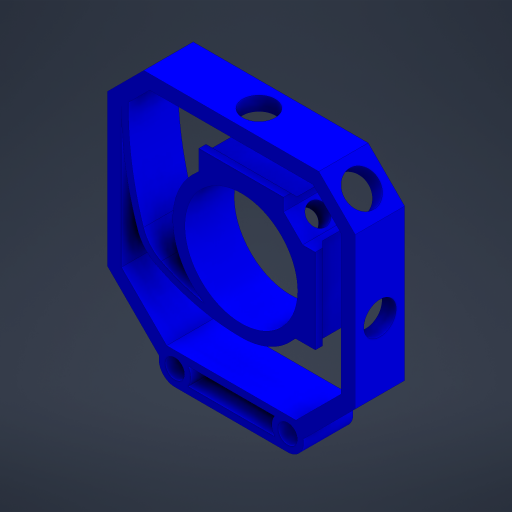
# Autodesk Inventor part: Laser Holder (USB)
Saved by Autodesk Inventor 2023.4 (Build 274418000, 418)
## iProperties
Created: 2022-07-25
Part Number: Laser Holder (USB)
Material: Generic
Document SubType Name: Modeling
Designer: xSibe
Density: 1 g/cm^3
Appearance: Plastic Blue
Author: xSibe
Autodesk Inventor part; units mm, degrees
ref_plane "YZ Plane" through (0, 0, 0) normal (1, 0, 0) x (0, 1, 0)
ref_plane "XZ Plane" through (0, 0, 0) normal (0, 1, 0) x (-1, 0, 0)
ref_plane "XY Plane" through (0, 0, 0) normal (0, 0, 1) x (1, 0, 0)
sketch "Sketch1" plane through (0, 0, 0) normal (0, 0, 1) x (1, 0, 0)
  circle A0 centre (10, 3.85) radius 1.5625 projected
  circle A1 centre (-10, 3.85) radius 1.5625 projected
  line L0 (-16.9, 0) -> (16.9, 0) projected
  line L1 (16.9, 0) -> (16.9, 7.7) projected
  line L2 (-16.9, 7.7) -> (16.9, 7.7) projected
  line L3 (-16.9, 0) -> (-16.9, 7.7) projected
  circle A2 centre (-10, 3.85) radius 2.8125
  circle A3 centre (10, 3.85) radius 2.8125
  line L4 (-10, 6.6625) -> (10, 6.6625)
  line L5 (10, 1.0375) -> (-10, 1.0375)
  line L6 (-10, 2.2875) -> (10, 2.2875)
  line L7 (-10, 5.4125) -> (10, 5.4125)
  line L8 (-17.05, 7.7) -> (-17.05, 42.1) projected
  line L9 (17.05, 7.7) -> (17.05, 42.1) projected
  line L10 (-17.05, 24.9) -> (17.05, 24.9)
  line L11 (0, 24.9) -> (1.7678, 26.6678)
  line L12 (0, 24.9) -> (2.5, 24.9) construction
  circle A4 centre (1.7678, 26.6678) radius 10
  circle A5 centre (1.7678, 26.6678) radius 7.5
  circle A6 centre (1.7678, 26.6678) radius 12.125
  line L13 (1.7678, 26.6678) -> (1.7678, 38.7928)
  line L14 (1.7678, 38.7928) -> (1.7678, 37.7928)
  line L15 (-5.7322, 35.7928) -> (9.2678, 35.7928)
  line L16 (9.2678, 35.7928) -> (9.2678, 39.7928)
  line L17 (9.2678, 39.7928) -> (-5.7322, 39.7928)
  line L18 (-5.7322, 39.7928) -> (-5.7322, 35.7928)
  line L19 (-5.7322, 35.7928) -> (9.2678, 39.7928) construction
  line L20 (9.2678, 35.7928) -> (-5.7322, 39.7928) construction
  line L21 (1.7678, 26.6678) -> (10.3414, 35.2414)
  line L22 (10.3414, 35.2414) -> (9.8995, 34.7995)
  line L23 (12.7279, 34.0924) -> (9.1924, 37.6279)
  line L24 (9.1924, 37.6279) -> (7.0711, 35.5066)
  line L25 (7.0711, 35.5066) -> (10.6066, 31.9711)
  line L26 (10.6066, 31.9711) -> (12.7279, 34.0924)
  line L27 (12.7279, 34.0924) -> (7.0711, 35.5066) construction
  line L28 (9.1924, 37.6279) -> (10.6066, 31.9711) construction
  line L29 (12.7279, 34.0924) -> (17.7279, 34.0924) construction
  line L30 (10.8928, 19.1678) -> (10.8928, 34.1678)
  line L31 (10.8928, 34.1678) -> (14.8928, 34.1678)
  line L32 (14.8928, 34.1678) -> (14.8928, 19.1678)
  line L33 (14.8928, 19.1678) -> (10.8928, 19.1678)
  line L34 (1.7678, 38.7928) -> (1.7678, 40.7928)
  line L35 (14.8928, 26.6678) -> (16.8928, 26.6678)
  line L36 (-10.2178, 5.4322) -> (10.2178, 5.4322)
  line L37 (19.4678, 14.6822) -> (19.4678, 39.3678)
  line L38 (14.4678, 44.3678) -> (-14.4678, 44.3678)
  line L39 (-19.4678, 39.3678) -> (-19.4678, 14.6822)
  line L40 (-19.4678, 5.4322) -> (19.4678, 44.3678) construction
  line L41 (19.4678, 5.4322) -> (-19.4678, 44.3678) construction
  line L42 (-10.2178, 5.4322) -> (-19.4678, 14.6822)
  line L43 (10.2178, 5.4322) -> (19.4678, 14.6822)
  line L44 (14.4678, 44.3678) -> (19.4678, 39.3678)
  line L45 (-14.4678, 44.3678) -> (-19.4678, 39.3678)
  line L46 (-15.5033, 46.8678) -> (-21.9678, 40.4033)
  line L47 (-21.9678, 40.4033) -> (-21.9678, 13.6467)
  line L48 (-21.9678, 13.6467) -> (-11.2533, 2.9322)
  line L49 (-11.2533, 2.9322) -> (11.2533, 2.9322)
  line L50 (11.2533, 2.9322) -> (21.9678, 13.6467)
  line L51 (21.9678, 13.6467) -> (21.9678, 40.4033)
  line L52 (21.9678, 40.4033) -> (15.5033, 46.8678)
  line L53 (15.5033, 46.8678) -> (-15.5033, 46.8678)
  circle A7 centre (-10, 3.85) radius 1.705
  circle A8 centre (10, 3.85) radius 1.707
  line L54 (1.7678, 14.5428) -> (-15.7322, 14.5428)
  line L55 (-15.7322, 14.5428) -> (-15.7322, 19.5428)
  arc A9 (-15.7322, 19.5428) -> (1.7678, 14.5428) centre (1.7678, 47.6678) ccw
  arc A10 (-19.4678, 39.3678) -> (-15.7322, 19.5428) centre (35.007, 39.3678) ccw
  arc A11 (-18.2027, 40.6328) -> (-14.7184, 20.3874) centre (35.007, 39.3678) ccw
  arc A12 (-14.7184, 20.3874) -> (-4.8026, 16.4773) centre (1.7678, 47.6678) ccw
  line L56 (-14.7184, 20.3874) -> (-15.5549, 22.7433)
  line L57 (-15.7322, 19.5428) -> (-16.5884, 21.8916)
  arc A13 (-15.5549, 22.7433) -> (-12.4238, 19.1263) centre (-9.6619, 24.6809) ccw
  arc A14 (-16.5884, 21.8916) -> (-13.459, 18.2499) centre (-10.5081, 23.9511) ccw
  line L58 (-10, 6.6625) -> (-11.448, 6.6625)
  line L59 (10, 6.6625) -> (11.448, 6.6625)
  point P0 (0, 0)
  point P1 (-7.6615, 2.2875)
  point P2 (-7.6615, 5.4125)
  point P3 (7.6615, 5.4125)
  point P4 (7.6615, 2.2875)
  point P5 (7.3415, 2.9322)
  point P6 (-7.3415, 2.9322)
  point P7 (-11.1858, 6.4003)
  point P8 (11.1858, 6.4003)
  point P9 (-5.7322, 36.1949)
  point P10 (11.2949, 19.1678)
  point P11 (11.2949, 34.1678)
  point P12 (11.925, 33.2894)
  point P13 (8.3894, 36.825)
  point P14 (9.2678, 36.1949)
  point P15 (12.7519, 4.4308)
  point P16 (-12.7519, 4.4308)
  point P17 (7.3572, 35.7928)
  point P18 (10.8928, 32.2572)
  point P19 (13.8928, 26.6678)
  point P20 (12.5533, 33.9178)
  point P21 (9.0178, 37.4533)
  point P22 (1.7678, 38.7928)
  point P23 (10.3414, 35.2414)
  point P24 (12.6525, 34.1678)
  point P25 (9.2678, 37.5525)
  point P26 (-5.6062, 36.2928)
  point P27 (11.3928, 19.2938)
  point P28 (11.3928, 34.0417)
  point P29 (9.1417, 36.2928)
  dimension "d0" = 1.25
  dimension "d1" = 1.25
  dimension "d2" = 2.5
  dimension "d3" = 45
  dimension "d4" = 20
  dimension "d5" = 2.5
  dimension "d6" = 2.125
  dimension "d7" = 1
  dimension "d8" = 15
  dimension "d9" = 4
  dimension "d10" = 0.625
  dimension "d11" = 5
  dimension "d12" = 135
  dimension "d13" = 3
  dimension "d14" = 2
  dimension "d15" = 2
  dimension "d16" = 38.9355
  dimension "d17" = 38.9355
  dimension "d18" = 9.25
  dimension "d19" = 9.25
  dimension "d20" = 9.25
  dimension "d21" = 9.25
  dimension "d22" = 5
  dimension "d23" = 5
  dimension "d24" = 5
  dimension "d25" = 5
  dimension "d26" = 2.5
  dimension "d46" = 0.1425
  dimension "d47" = 0.1445
  dimension "d48" = 17.5
  dimension "d49" = 5
  dimension "d50" = 1.25
  dimension "d51" = 2.5
  dimension "d52" = 2.5
  constraints: 108 end point, 29 point on circle, 18 point on line, 13 centre point, 13 tangent, 10 midpoint, 8 parallel, 7 horizontal, 7 perpendicular, 4 symmetric about line, 2 equal length, 1 coincident, 1 vertical, 8 other
  measures "d0" radial gap between concentric circles of A1 A2
  measures "d1" radial gap between concentric circles of A0 A3
  measures "d2" distance of L11.start L11.end
  measures "d3" angle of L12 L11
  measures "d4" diameter of A4
  measures "d5" radial gap between concentric circles of A4 A5
  measures "d6" radial gap between concentric circles of A4 A6
  measures "d7" distance of L13.end L14.end
  measures "d8" distance of L17.end L16.end
  measures "d9" distance of L16.end L15.end
  measures "d10" distance of L21.end L22.end
  measures "d11" distance of L23.start L23.end
  measures "d12" angle of L29 L23
  measures "d13" distance of L24.end L23.end
  measures "d14" distance of L13.end L34.end
  measures "d15" distance of L35.start L35.end
  measures "d16" distance of L40.end L41.end
  measures "d17" distance of L41.end L40.start
  measures "d18" distance of L36.start L40.start
  measures "d19" distance of L39.end L40.start
  measures "d20" distance of L36.end L41.start
  measures "d21" distance of L37.start L41.start
  measures "d22" distance of L38.start L40.end
  measures "d23" distance of L37.end L40.end
  measures "d24" distance of L38.end L41.end
  measures "d25" distance of L39.start L41.end
  measures "d26" distance between parallel lines of L38 L53
  measures "d46" radial gap between concentric circles of A1 A7
  measures "d47" radial gap between concentric circles of A0 A8
  measures "d48" distance of L54.start L54.end
  measures "d49" distance of L54.end L55.end
  measures "d50" radial gap between concentric circles of A10 A11
  measures "d51" distance of L56.start L56.end
  measures "d52" distance of L55.end L57.end
extrude "Extrusion1" add sketch "Sketch1" along normal mid plane 8.75 contours A8 L49 A3 L7 | L7 A3 L36 A8 | A8 L43 A3 L50 | L50 A3 L6 A8 | A8 L6 A3 L49 | L7 A2 L36 A3 | L36 A3 L43 A8 | A3 L43 L2 L50 | L36 A2 L4 A3 | L7 A7 L36 A2 | A2 L49 A7 L7 | A3 L5 A2 L6 | A3 L59 L43 | L2 L43 L9 L50 | A2 L6 A7 L49 | L36 A7 L42 A2 | A2 L48 A7 L6 | L9 L43 L37 L44 L38 L45 L39 L42 L8 L48 L47 L46 L53 L52 L51 L50 | A2 L42 L58 | L42 A2 L48 L2 | L2 L48 L8 L42 | L42 A7 L48 A2 | A10 L45 A11 L8 | L8 L10 A11 A12 A6 A9 A14 A10 | L32 L33 A6 L10 | L10 A6 L26 L23 L31 L32 | L8 A11 L10 | A6 L33 L30 A4 L10 | L10 A4 L30 L26 A6 | A13 A12 L56 | A6 L10 A4 L30 L33 | A6 L18 L15 A4 L10 | L56 A11 | L26 L30 L31 A6 | A6 L31 L23 L26 | L31 A6 L16 L23 | L18 L17 L34 A6 | A6 L13 A4 L15 L18 | A4 L25 L26 L30 | L31 L30 L26 L25 L21 A6 | L23 L24 A6 L34 L17 L16 | L16 A6 L24 L23 | A6 L24 L15 A4 L13 | L25 L24 L15 L16 A6 L21 | A4 L15 L24 L25 | L16 L15 L24 A6
sketch "Sketch2" plane through (0, 0, 0) normal (0, 0, 1) x (1, 0, 0)
  circle A0 centre (1.7678, 26.6678) radius 10 projected
  circle A1 centre (1.7678, 26.6678) radius 8.125
  point P0 (0, 0)
  dimension "d30" = 1.875
  constraints: 1 centre point
  measures "d30" radial gap between concentric circles of A0 A1
extrude "Extrusion2" [suppressed]
sketch "Sketch3" plane through (21.9678, 13.6467, -4.375) normal (1, 0, 0) x (0, 0, -1)
  line L0 (0, 5.5211) -> (-8.75, 5.5211) projected
  line L1 (0, 20.5211) -> (0, 5.5211) projected
  line L2 (-8.75, 5.5211) -> (-8.75, 20.5211) projected
  line L3 (-4.375, 18.0211) -> (-4.375, 5.5211)
  circle A0 centre (-4.375, 11.7711) radius 2.875
  line L4 (0, 20.5211) -> (-8.75, 20.5211) projected
  point P0 (-4.375, -13.6467)
  dimension "d33" = 5.75
  constraints: 2 end point, 2 midpoint, 1 centre point
  measures "d33" diameter of A0
extrude "Extrusion3" cut sketch "Sketch3" against normal up to surface (2.5 mm away) contours A0 L3 | L3 A0
sketch "Sketch4" plane through (12.2614, 34.1678, -4.375) normal (0, 1, 0) x (1, 0, 0)
  line L0 (2.6314, 0) -> (2.6314, -8.75) projected
  line L1 (0.3912, 0) -> (2.6314, 0) projected
  line L2 (2.6314, -8.75) -> (0.3912, -8.75) projected
  line L3 (2.6314, -8.75) -> (0.3912, -8.75)
  line L4 (0.3912, -8.75) -> (0.3912, -7.5)
  line L5 (0.3912, -7.5) -> (2.6314, -7.5)
  line L6 (2.6314, -7.5) -> (2.6314, -8.75)
  line L7 (2.6314, -7.5) -> (0.3912, -5.2598)
  line L8 (2.6314, -7.5) -> (5.7996, -7.5) construction
  line L9 (0.3912, -4.375) -> (2.6314, -4.375)
  line L10 (2.6314, -1.25) -> (0.3912, -3.4902)
  line L11 (1.5113, -8.75) -> (1.5113, 0)
  line L12 (0.3912, 0) -> (0.3912, -8.75) projected
  point P0 (-12.2614, -4.375)
  point P1 (2.6314, -1.25)
  point P2 (2.6314, -7.5)
  point P3 (1.5113, -2.3701)
  point P4 (1.5113, -6.3799)
  dimension "d36" = 1.25
  dimension "d37" = 135
  constraints: 18 end point, 4 midpoint, 2 horizontal, 2 parallel, 2 symmetric about line, 1 equal length, 1 perpendicular, 1 point on line
  measures "d36" distance of L2.end L4.end
  measures "d37" angle of L8 L7
extrude "Extrusion4" cut sketch "Sketch4" against normal up to surface (15 mm away) contours L0 L9 L11 L10 | L0 L7 L11 L9
ref_plane "Work Plane1" through (14.8928, 39.7928, 4.375) normal (0.7071068, -0.7071068, 0) x (0, 0, -1)
mirror "Mirror1" about plane through (14.8928, 39.7928, 4.375) normal (0.7071068, -0.7071068, 0) of "Extrusion3", "Extrusion4"
sketch "Sketch5" plane through (21.9678, 40.4033, 4.375) normal (0.7071068, 0.7071068, 0) x (0.7071068, -0.7071068, 0)
  line L0 (0, 8.75) -> (0, 0) projected
  line L1 (-9.1421, 8.75) -> (0, 8.75) projected
  line L2 (-9.1421, 8.75) -> (-9.1421, 0) projected
  line L3 (0, 0) -> (-9.1421, 0) projected
  line L4 (-6.9645, 8.75) -> (-2.1777, 8.75) projected
  line L5 (-2.1777, 0) -> (-6.9645, 0) projected
  circle A0 centre (-4.5711, 4.375) radius 1.875
  line L6 (-7.0711, 4.375) -> (-2.0711, 4.375)
  circle A1 centre (-4.5711, 4.375) radius 3
  line L7 (-6.9645, 8.75) -> (-6.9645, 0) projected
  line L8 (-2.1777, 8.75) -> (-2.1777, 0) projected
  point P0 (13.0359, 4.375)
  dimension "d40" = 3.75
  dimension "d41" = 6
  constraints: 2 centre point, 2 end point, 1 coincident, 1 midpoint
  measures "d40" diameter of A0
  measures "d41" diameter of A1
extrude "Extrusion5" cut sketch "Sketch5" against normal up to surface (2.5 mm away) contours L8 L6 A0 L7 A1 | A1 L8 | A1 L7 L6 A0 L8 | L7 A1 | L6 A0 | A0 L6
extrude "Extrusion6" cut sketch "Sketch5" against normal up to surface from surface at -10.996 contours L6 A0 | A0 L6 round surface about axis through (1.7678, 26.6678, 0) along (0, 0, 1) radius 10 far side no
equation "\"d19\" = d18"
equation "\"d20\" = d18"
equation "\"d21\" = d20"
equation "\"d23\" = d22"
equation "\"d24\" = d22"
equation "\"d25\" = d24"
body "Solid1"
